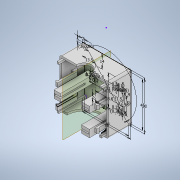
# Autodesk Inventor part: Light_PCB_Holder
Saved by Autodesk Inventor 2022 (Build 260153000, 153)
## iProperties
Created: 2022-08-01
Part Number: Light_PCB_Holder
Material: Generic
Document SubType Name: Modeling
Designer: sgioj
Density: 1 g/cm^3
Appearance: Default
Author: sgioj
Autodesk Inventor part; units mm, degrees
ref_plane "YZ Plane" through (0, 0, 0) normal (1, 0, 0) x (0, 1, 0)
ref_plane "XZ Plane" through (0, 0, 0) normal (0, 1, 0) x (-1, 0, 0)
ref_plane "XY Plane" through (0, 0, 0) normal (0, 0, 1) x (1, 0, 0)
sketch "Sketch1" plane through (0, 0, 0) normal (0, 0, 1) x (1, 0, 0)
  line L0 (0, 0) -> (50, 0)
  line L1 (50, 0) -> (50, -50)
  line L2 (50, -50) -> (0, -50)
  line L3 (0, -50) -> (0, 0)
  line L4 (13.5, -14) -> (34.5, -14) construction
  line L5 (34.5, -14) -> (34.5, -45) construction
  line L6 (34.5, -45) -> (13.5, -45) construction
  line L7 (13.5, -45) -> (13.5, -14) construction
  line L8 (2, -2) -> (48, -2)
  line L9 (48, -2) -> (48, -48)
  line L10 (48, -48) -> (2, -48)
  line L11 (2, -48) -> (2, -2)
  line L12 (13.5, -21.5) -> (34.5, -21.5) construction
  line L13 (34.5, -21.5) -> (34.5, -43) construction
  line L14 (34.5, -43) -> (13.5, -43) construction
  line L15 (13.5, -43) -> (13.5, -21.5) construction
  line L16 (13.5, -43) -> (42.1, -43) construction
  line L17 (42.1, -43) -> (42.1, -42) construction
  line L18 (42.1, -42) -> (13.5, -42) construction
  line L19 (13.5, -42) -> (13.5, -43) construction
  line L20 (42.1, -25) -> (7.3, -25) construction
  line L21 (7.3, -25) -> (7.3, -26) construction
  line L22 (7.3, -26) -> (42.1, -26) construction
  line L23 (42.1, -26) -> (42.1, -25) construction
  line L24 (13.5, -21.5) -> (42.1, -21.5) construction
  line L25 (42.1, -21.5) -> (42.1, -22.5) construction
  line L26 (42.1, -22.5) -> (13.5, -22.5) construction
  line L27 (13.5, -22.5) -> (13.5, -21.5) construction
  line L28 (34.75, -22.8) -> (42.85, -22.8)
  line L29 (42.85, -22.8) -> (42.85, -24.7)
  line L30 (42.85, -24.7) -> (34.75, -24.7)
  line L31 (34.75, -24.7) -> (34.75, -22.8)
  line L32 (42.85, -22.8) -> (42.35, -22.8)
  line L33 (42.35, -22.8) -> (42.35, -18.2)
  line L34 (42.35, -18.2) -> (42.85, -18.2)
  line L35 (42.85, -18.2) -> (42.85, -22.8)
  line L36 (42.85, -21.2) -> (34.75, -21.2)
  line L37 (34.75, -21.2) -> (34.75, -18.2)
  line L38 (34.75, -18.2) -> (42.85, -18.2)
  line L39 (42.85, -18.2) -> (42.85, -21.2)
  line L40 (13.2, -24.7) -> (13.2, -21.7)
  line L41 (13.2, -24.7) -> (7.05, -24.7)
  line L42 (7.05, -24.7) -> (7.05, -26.3)
  line L43 (7.05, -26.3) -> (13.2, -26.3)
  line L44 (13.2, -26.3) -> (13.2, -29.3)
  line L45 (13.2, -29.3) -> (6.55, -29.3)
  line L46 (6.55, -29.3) -> (6.55, -21.7)
  line L47 (6.55, -21.7) -> (13.2, -21.7)
  line L48 (34.75, -41.7) -> (42.35, -41.7)
  line L49 (42.35, -41.7) -> (42.35, -43.3)
  line L50 (42.35, -43.3) -> (34.75, -43.3)
  line L51 (34.75, -43.3) -> (34.75, -46.3)
  line L52 (34.75, -46.3) -> (42.85, -46.3)
  line L53 (42.85, -46.3) -> (42.85, -38.7)
  line L54 (42.85, -38.7) -> (34.75, -38.7)
  line L55 (34.75, -38.7) -> (34.75, -41.7)
  line L56 (25, 0) -> (25, -57.0904) construction
  line L57 (2.2, -2.2) -> (4.2, -2.2)
  line L58 (4.2, -2.2) -> (4.2, -4.2)
  line L59 (4.2, -4.2) -> (2.2, -4.2)
  line L60 (2.2, -4.2) -> (2.2, -2.2)
  line L61 (2.2, -45.8) -> (4.2, -45.8)
  line L62 (2.2, -47.8) -> (2.2, -45.8)
  line L63 (4.2, -47.8) -> (2.2, -47.8)
  line L64 (4.2, -45.8) -> (4.2, -47.8)
  line L65 (45.8, -47.8) -> (45.8, -45.8)
  line L66 (47.8, -47.8) -> (45.8, -47.8)
  line L67 (47.8, -45.8) -> (47.8, -47.8)
  line L68 (45.8, -45.8) -> (47.8, -45.8)
  line L69 (47.8, -4.2) -> (45.8, -4.2)
  line L70 (47.8, -2.2) -> (47.8, -4.2)
  line L71 (45.8, -2.2) -> (47.8, -2.2)
  line L72 (45.8, -4.2) -> (45.8, -2.2)
  line L73 (13.2, -24.7) -> (13.2, -26.3)
  line L74 (34.75, -21.2) -> (34.75, -22.8)
  line L75 (34.75, -41.7) -> (34.75, -43.3)
  point P0 (42.35, -21.2)
  point P1 (25, 25)
  point P2 (25, -25)
  dimension "d0" = 50
  dimension "d1" = 50
  dimension "d2" = 21
  dimension "d3" = 31
  dimension "d4" = 14
  dimension "d5" = 46
  dimension "d6" = 46
  dimension "d7" = 2
  dimension "d8" = 2
  dimension "d9" = 13.5
  dimension "d10" = 21
  dimension "d11" = 21.5
  dimension "d12" = 28.6
  dimension "d13" = 1
  dimension "d14" = 34.8
  dimension "d15" = 1
  dimension "d16" = 18
  dimension "d17" = 1
  dimension "d18" = 21.5
  dimension "d19" = 2
  dimension "d21" = 1.9
  dimension "d22" = 0.3
  dimension "d23" = 0.25
  dimension "d24" = 0.5
  dimension "d25" = 28.6
  dimension "d26" = 0.25
  dimension "d27" = 3
  dimension "d28" = 0
  dimension "d29" = 1.6
  dimension "d30" = 0.3
  dimension "d31" = 0.25
  dimension "d32" = 8.1
  dimension "d33" = 0
  dimension "d34" = 8.1
  dimension "d35" = 3
  dimension "d36" = 3
  dimension "d37" = 0.3
  dimension "d38" = 0.3
  dimension "d39" = 0.3
  dimension "d40" = 0.3
  dimension "d41" = 0.5
  dimension "d42" = 0.25
  dimension "d43" = 0.3
  dimension "d44" = 0.3
  dimension "d45" = 0.25
  dimension "d46" = 0.25
  dimension "d47" = 0.25
  dimension "d48" = 3
  dimension "d49" = 0.5
  dimension "d50" = 3
  dimension "d88" = 2
  dimension "d89" = 2
  dimension "d92" = 360
  constraints: 152 end point, 25 parallel, 23 perpendicular, 12 horizontal, 5 point on line, 2 vertical, 1 midpoint, 33 other
  measures "d0" distance of L1.end L2.end
  measures "d1" distance of L0.end L1.end
  measures "d2" distance of L5.end L6.end
  measures "d3" distance of L4.end L5.end
  measures "d4" distance between parallel lines of L0 L4
  measures "d5" distance of L9.end L10.end
  measures "d6" distance of L8.end L9.end
  measures "d7" distance between parallel lines of L0 L8
  measures "d8" distance between parallel lines of L11 L3
  measures "d9" distance between parallel lines of L3 L7
  measures "d10" distance of L13.end L14.end
  measures "d11" distance of L12.end L13.end
  measures "d12" distance of L18.end L17.end
  measures "d13" distance of L17.end L16.end
  measures "d14" distance of L22.end L21.end
  measures "d15" distance of L21.end L20.end
  measures "d16" distance between parallel lines of L20 L16
  measures "d17" distance of L24.end L25.end
  measures "d18" distance between parallel lines of L16 L24
  measures "d19" distance between parallel lines of L16 L6
  measures "d21" distance of L28.end L29.end
  measures "d22" distance between parallel lines of L26 L28
  measures "d23" distance between parallel lines of L13 L31
  measures "d24" distance between parallel lines of L35 L33
  measures "d25" distance between parallel lines of L15 L25
  measures "d26" distance between parallel lines of L25 L33
  measures "d27" distance of L36.end L37.end
  measures "d28" distance between parallel lines of L38 L34
  measures "d29" distance between parallel lines of L36 L28
  measures "d30" distance between parallel lines of L30 L20
  measures "d31" distance between parallel lines of L5 L37
  measures "d32" distance between parallel lines of L35 L37
  measures "d33" distance between parallel lines of L7 L15
  measures "d34" distance between parallel lines of L29 L31
  measures "d35" distance of L40.start L40.end
  measures "d36" distance of L43.end L44.end
  measures "d37" distance between parallel lines of L41 L20
  measures "d38" distance between parallel lines of L22 L43
  measures "d39" distance between parallel lines of L7 L40
  measures "d40" distance between parallel lines of L7 L44
  measures "d41" distance between parallel lines of L46 L42
  measures "d42" distance between parallel lines of L42 L21
  measures "d43" distance between parallel lines of L16 L50
  measures "d44" distance between parallel lines of L48 L18
  measures "d45" distance between parallel lines of L49 L17
  measures "d46" distance between parallel lines of L13 L55
  measures "d47" distance between parallel lines of L5 L51
  measures "d48" distance between parallel lines of L48 L54
  measures "d49" distance between parallel lines of L53 L49
  measures "d50" distance between parallel lines of L52 L50
  measures "d88" distance of L58.end L59.end
  measures "d89" distance of L57.end L58.end
extrude "Extrusion1" add sketch "Sketch1" along normal blind 23 contours L0 L1 L2 L3
extrude "Extrusion2" add sketch "Sketch1" against normal blind 2 contours L0 L1 L2 L3 | L8 L9 L10 L11 | L74 L36 L33 L28 | L28 L29 L30 L31 | L33 L36 L35 L28 | L37 L38 L33 L36 | L33 L34 L35 L36 | L41 L42 L43 L44 L45 L46 L47 L40 | L73 L43 L42 L41 | L55 L54 L53 L52 L51 L50 L49 L48 | L48 L49 L50 L75 | L57 L58 L59 L60 | L61 L64 L63 L62 | L65 L68 L67 L66 | L69 L72 L71 L70
sketch "Sketch2" plane through (0, -50, 23) normal (0, -1, 0) x (1, 0, 0)
  line L0 (0, 0) -> (50, 0) projected
  circle A0 centre (25, 0) radius 17.5
  point P0 (0, -23)
  point P1 (42.5, 0)
  point P2 (7.5, 0)
  dimension "d55" = 35
  constraints: 1 centre point, 1 midpoint
  measures "d55" diameter of A0
extrude "Extrusion3" cut sketch "Sketch2" against normal blind 2 contours L0 A0 picked at (19.8348, -2.7109)
sketch "Sketch3" plane through (0, 0, 23) normal (0, 1, 0) x (1, 0, 0)
  line L0 (50, 0) -> (0, 0) projected
  circle A0 centre (25, 0) radius 7.5
  point P0 (0, 23)
  point P1 (17.5, 0)
  point P2 (32.5, 0)
  dimension "d58" = 15
  constraints: 1 centre point, 1 midpoint
  measures "d58" diameter of A0
extrude "Extrusion4" cut sketch "Sketch3" against normal blind 2 contours L0 A0 picked at (22.5, 3.3156)
sketch "Sketch4" plane through (2, -48, 23) normal (1, 0, 0) x (0, 0, -1)
  line L0 (10, 5) -> (15, 5)
  line L1 (15, 5) -> (15, 9)
  line L2 (15, 9) -> (10, 9)
  line L3 (10, 9) -> (10, 5)
  line L4 (0, 0) -> (0, 46) projected
  line L5 (23, 0) -> (0, 0) projected
  point P0 (23, 48)
  dimension "d61" = 5
  dimension "d62" = 4
  dimension "d80" = 10
  dimension "d81" = 5
  constraints: 8 end point, 2 parallel, 1 horizontal, 1 perpendicular
  measures "d61" distance of L2.end L1.end
  measures "d62" distance of L1.end L0.end
  measures "d80" distance between parallel lines of L4 L3
  measures "d81" distance between parallel lines of L5 L0
extrude "Extrusion5" add sketch "Sketch4" along normal blind 4
sketch "Sketch5" plane through (2, -43, 13) normal (0, 0, 1) x (1, 0, 0)
  line L0 (0, 4) -> (4, 4) projected
  line L1 (4, 4) -> (2, 4)
  line L2 (2, 4) -> (2, 0)
  line L3 (2, 0) -> (4, 0)
  line L4 (4, 0) -> (4, 4)
  point P0 (-2, 43)
  point P1 (2, 4)
  dimension "d67" = 2
  dimension "d82" = 4
  constraints: 8 end point, 2 parallel, 1 horizontal, 1 perpendicular
  measures "d67" distance of L3.end L2.end
  measures "d82" distance between parallel lines of L0 L3
extrude "Extrusion6" add sketch "Sketch5" along normal blind 18
sketch "Sketch6" plane through (2, -43, 8) normal (0, -1, 0) x (1, 0, 0)
  line L0 (2, 23) -> (4, 23) projected
  line L1 (2, 23) -> (0.7272, 21.7272)
  line L2 (2, 23) -> (3.8, 23) construction
  line L3 (0.7272, 21.7272) -> (2, 20.4544)
  line L4 (2, 5) -> (2, 23) projected
  point P0 (-2, -8)
  dimension "d70" = 1.8
  dimension "d71" = 135
  dimension "d72" = 1.8
  constraints: 6 end point, 1 equal length, 1 horizontal, 1 point on line
  measures "d70" distance of L0.start L1.end
  measures "d71" angle of L1 L2
  measures "d72" distance of L1.end L3.end
extrude "Extrusion7" add sketch "Sketch6" against normal blind 4
chamfer "Chamfer1" distance 3 angle 45 1 edges at (6, -41, 8)
extrude "Extrusion8" add sketch "Sketch1" along normal blind 35.4 contours L28 L29 L30 L31 | L33 L36 L35 L28 | L37 L38 L33 L36 | L33 L34 L35 L36 | L41 L42 L43 L44 L45 L46 L47 L40 | L55 L54 L53 L52 L51 L50 L49 L48
sketch "Sketch7" plane through (2, -39, 13) normal (0, 1, 0) x (1, 0, 0)
  line L0 (4, -18) -> (2, -18) projected
  line L1 (4, -18) -> (2, -18)
  line L2 (0.7272, -16.7272) -> (2, -18) projected
  line L3 (2, -18) -> (0.7272, -16.7272)
  line L4 (0.7272, -16.7272) -> (2, -15.4544)
  line L5 (2, -15.4544) -> (2, 0)
  line L6 (0, 0) -> (0, 5) projected
  line L7 (2, 0) -> (0, 0)
  line L8 (0, 5) -> (1, 5) projected
  line L9 (0, 0) -> (0, 5)
  line L10 (0, 5) -> (1, 5)
  line L11 (1, 5) -> (4, 2) projected
  line L12 (1, 5) -> (4, 2)
  line L13 (4, 2) -> (4, -18)
  point P0 (-2, 13)
  constraints: 18 end point, 5 perpendicular, 3 collinear, 1 parallel
pattern_linear "Rectangular Pattern1" count 2 spacing 21 along (0, 1, 0) of "Extrusion5", "Extrusion6", "Chamfer1", "Extrusion7"
ref_plane "Work Plane1" through (25, 0, 0) normal (-1, 0, 0) x (0, -1, 0)
mirror "Mirror1" about plane through (25, 0, 0) normal (-1, 0, 0) of "Extrusion5", "Extrusion6", "Chamfer1", "Extrusion7", "Rectangular Pattern1"
fillet "Fillet1" radius 2 8 edges at (0, -50, 10.5) (50, -50, 10.5) (25, -50, -2) (0, -25, -2) (50, -25, -2) (25, 0, -2) (0, 0, 10.5) (50, 0, 10.5)
extrude "Extrusion9" add sketch "Sketch1" along normal blind 28 contours L57 L58 L59 L60 | L61 L64 L63 L62 | L65 L68 L67 L66 | L69 L72 L71 L70
extrude "Extrusion10" add sketch "Sketch1" along normal blind 10.2 contours L74 L36 L33 L28 | L73 L43 L42 L41 | L48 L49 L50 L75
extrude "Extrusion11" add sketch "Sketch1" along normal blind 12 contours L48 L49 L50 L75
body "Solid1"
